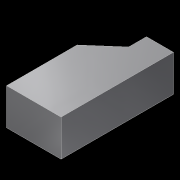
# Autodesk Inventor part: Part1
Saved by Autodesk Inventor 2021.1 (Build 251245000, 245)
## iProperties
Created: 2020-08-29
Part Number: Part1
Material: A5052
Document SubType Name: Modeling
Designer: Hashimoto
Mass: 5.10202 g
Surface Area: 13.3196 cm^2
Volume: 1.88237 cm^3
Density: 2.71043 g/cm^3
Appearance: アルミニウム - つや出し
Author: Hashimoto
Autodesk Inventor part; units mm, degrees
ref_plane "YZ Plane" through (0, 0, 0) normal (1, 0, 0) x (0, 1, 0)
ref_plane "XZ Plane" through (0, 0, 0) normal (0, 1, 0) x (-1, 0, 0)
ref_plane "XY Plane" through (0, 0, 0) normal (0, 0, 1) x (1, 0, 0)
sketch "スケッチ22" plane through (0, 0, 0) normal (0, 0, 1) x (1, 0, 0)
  line L0 (-7.557, -9.0332) -> (-7.557, 10.3172)
  line L1 (-7.557, 10.3172) -> (0, 16.9371)
  line L2 (0, 16.9371) -> (0, 21.8256)
  line L3 (0, 21.8256) -> (7.4141, 21.8256)
  line L4 (7.4141, 21.8256) -> (7.4141, -9.0332)
  line L5 (7.4141, -9.0332) -> (-7.557, -9.0332)
  point P0 (0, 0)
  constraints: 12 end point, 3 perpendicular, 1 parallel, 1 vertical
extrude "押し出し14" add sketch "スケッチ22" along normal blind 5
sketch "スケッチ23" plane through (0, 0, 5) normal (0, 0, 1) x (1, 0, 0)
  point P0 (0, 0)
  point P1 (3.7071, -4.7473)
  point P2 (-4.261, -4.7473)
hole "穴9" at (3.7071, -4.7473, 5) at (-4.261, -4.7473, 5) direction (0, 0, -1) diameter 5 depth 3
